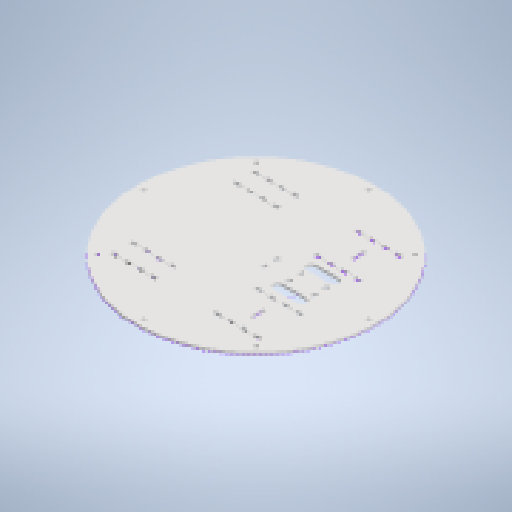
# Autodesk Inventor part: Osn. platform
Saved by Autodesk Inventor 2023.1 (Build 271208000, 208)
## iProperties
Created: 2023-03-13
Part Number: Osn. platform
Material: Типовые
Document SubType Name: Modeling
Designer: User
Density: 1 g/cm^3
Appearance: По умолчанию
Author: User
Autodesk Inventor part; units mm, degrees
ref_plane "YZ Plane" through (0, 0, 0) normal (1, 0, 0) x (0, 1, 0)
ref_plane "XZ Plane" through (0, 0, 0) normal (0, 1, 0) x (-1, 0, 0)
ref_plane "XY Plane" through (0, 0, 0) normal (0, 0, 1) x (1, 0, 0)
sketch "Основ. платформа" plane through (0, 0, 0) normal (0, 1, 0) x (-1, 0, 0)
  circle A0 centre (0, 0) radius 240
  dimension "d117" = 480
  constraints: 1 centre point, 1 coincident
  measures "d117" diameter of A0
extrude "Осн. платформа" add sketch "Основ. платформа" along normal blind 5
sketch "Эскиз14" plane through (0, 5, 0) normal (0, 1, 0) x (1, 0, 0)
  line L0 (-295.6598, 0) -> (443.256, 0) construction
  line L1 (137.6204, 61.9298) -> (150.9061, 61.9298)
  line L2 (150.9061, 61.9298) -> (150.9061, 55.9298)
  line L3 (137.6204, 55.9298) -> (150.9061, 55.9298)
  line L4 (137.6204, 61.9298) -> (137.6204, 55.9298)
  line L5 (111.049, 61.9298) -> (124.3347, 61.9298)
  line L6 (124.3347, 61.9298) -> (124.3347, 55.9298)
  line L7 (111.049, 55.9298) -> (124.3347, 55.9298)
  line L8 (111.049, 61.9298) -> (111.049, 55.9298)
  line L9 (84.4776, 61.9298) -> (97.7633, 61.9298)
  line L10 (97.7633, 61.9298) -> (97.7633, 55.9298)
  line L11 (84.4776, 55.9298) -> (97.7633, 55.9298)
  line L12 (84.4776, 61.9298) -> (84.4776, 55.9298)
  line L13 (57.9061, 144.9298) -> (71.1919, 144.9298)
  line L14 (71.1919, 144.9298) -> (71.1919, 138.9298)
  line L15 (57.9061, 138.9298) -> (71.1919, 138.9298)
  line L16 (57.9061, 144.9298) -> (57.9061, 138.9298)
  line L17 (84.4776, 144.9298) -> (97.7633, 144.9298)
  line L18 (97.7633, 144.9298) -> (97.7633, 138.9298)
  line L19 (84.4776, 138.9298) -> (97.7633, 138.9298)
  line L20 (84.4776, 144.9298) -> (84.4776, 138.9298)
  line L21 (111.049, 144.9298) -> (124.3347, 144.9298)
  line L22 (124.3347, 144.9298) -> (124.3347, 138.9298)
  line L23 (111.049, 138.9298) -> (124.3347, 138.9298)
  line L24 (111.049, 144.9298) -> (111.049, 138.9298)
  line L25 (137.6204, 144.9298) -> (150.9061, 144.9298)
  line L26 (150.9061, 144.9298) -> (150.9061, 138.9298)
  line L27 (137.6204, 138.9298) -> (150.9061, 138.9298)
  line L28 (137.6204, 144.9298) -> (137.6204, 138.9298)
  line L29 (101.4061, 87.5965) -> (101.4061, 113.2631)
  line L30 (101.4061, 113.2631) -> (107.4061, 113.2631)
  line L31 (107.4061, 113.2631) -> (107.4061, 87.5965)
  line L32 (107.4061, 87.5965) -> (101.4061, 87.5965)
  line L33 (57.9061, 61.9298) -> (71.1919, 61.9298)
  line L34 (71.1919, 61.9298) -> (71.1919, 55.9298)
  line L35 (57.9061, 55.9298) -> (71.1919, 55.9298)
  line L36 (57.9061, 61.9298) -> (57.9061, 55.9298)
  line L37 (-58.1024, 138.9298) -> (-70.9595, 138.9298)
  line L38 (-70.9595, 138.9298) -> (-70.9595, 144.9298)
  line L39 (-58.1024, 144.9298) -> (-70.9595, 144.9298)
  line L40 (-58.1024, 138.9298) -> (-58.1024, 144.9298)
  line L41 (-83.8167, 138.9298) -> (-96.6738, 138.9298)
  line L42 (-96.6738, 138.9298) -> (-96.6738, 144.9298)
  line L43 (-83.8167, 144.9298) -> (-96.6738, 144.9298)
  line L44 (-83.8167, 138.9298) -> (-83.8167, 144.9298)
  line L45 (-109.531, 138.9298) -> (-122.3881, 138.9298)
  line L46 (-122.3881, 138.9298) -> (-122.3881, 144.9298)
  line L47 (-109.531, 144.9298) -> (-122.3881, 144.9298)
  line L48 (-109.531, 138.9298) -> (-109.531, 144.9298)
  line L49 (-135.2452, 138.9298) -> (-148.1024, 138.9298)
  line L50 (-148.1024, 138.9298) -> (-148.1024, 144.9298)
  line L51 (-135.2452, 144.9298) -> (-148.1024, 144.9298)
  line L52 (-135.2452, 138.9298) -> (-135.2452, 144.9298)
  line L53 (-58.1024, 144.9298) -> (-148.1024, 144.9298) construction
  line L54 (-148.1024, 100.7298) -> (-58.1024, 100.7298) construction
  line L55 (137.6204, 138.9298) -> (124.3347, 144.9298) construction
  circle A0 centre (130.9776, 141.9298) radius 1.5
  circle A1 centre (104.2556, 141.9298) radius 1.5
  circle A2 centre (77.5336, 141.9298) radius 1.5
  circle A3 centre (130.9776, 58.9298) radius 1.5
  circle A4 centre (104.2556, 58.9298) radius 1.5
  circle A5 centre (77.5336, 58.9298) radius 1.5
  line L56 (-70.9595, 138.9298) -> (-83.8167, 144.9298) construction
  circle A6 centre (-77.3881, 141.9298) radius 1.5
  circle A7 centre (-103.2571, 141.9298) radius 1.5
  circle A8 centre (-129.1261, 141.9298) radius 1.5
  line L57 (-122.3881, 106.7298) -> (-122.3881, 100.7298)
  line L58 (-109.531, 100.7298) -> (-122.3881, 100.7298)
  line L59 (-109.531, 106.7298) -> (-109.531, 100.7298)
  line L60 (-109.531, 106.7298) -> (-122.3881, 106.7298)
  line L61 (-83.8167, 106.7298) -> (-96.6738, 106.7298)
  line L62 (-70.9595, 106.7298) -> (-70.9595, 100.7298)
  line L63 (-58.1024, 100.7298) -> (-70.9595, 100.7298)
  circle A9 centre (-103.2571, 103.7298) radius 1.5
  circle A10 centre (-129.1261, 103.7298) radius 1.5
  line L64 (-135.2452, 106.7298) -> (-135.2452, 100.7298)
  line L65 (-148.1024, 106.7298) -> (-148.1024, 100.7298)
  line L66 (-135.2452, 100.7298) -> (-148.1024, 100.7298)
  line L67 (-135.2452, 106.7298) -> (-148.1024, 106.7298)
  line L68 (-58.1024, 106.7298) -> (-70.9595, 106.7298)
  line L69 (-58.1024, 106.7298) -> (-58.1024, 100.7298)
  line L70 (-96.6738, 106.7298) -> (-96.6738, 100.7298)
  line L71 (-83.8167, 100.7298) -> (-96.6738, 100.7298)
  line L72 (-83.8167, 106.7298) -> (-83.8167, 100.7298)
  circle A11 centre (-77.3881, 103.7298) radius 1.5
  line L73 (111.049, -61.9298) -> (124.3347, -61.9298)
  line L74 (111.049, -61.9298) -> (111.049, -55.9298)
  line L75 (97.7633, -61.9298) -> (97.7633, -55.9298)
  line L76 (71.1919, -61.9298) -> (71.1919, -55.9298)
  line L77 (57.9061, -61.9298) -> (57.9061, -55.9298)
  line L78 (57.9061, -55.9298) -> (71.1919, -55.9298)
  line L79 (57.9061, -61.9298) -> (71.1919, -61.9298)
  line L80 (107.4061, -87.5965) -> (101.4061, -87.5965)
  line L81 (101.4061, -87.5965) -> (101.4061, -113.2631)
  line L82 (107.4061, -113.2631) -> (107.4061, -87.5965)
  line L83 (57.9061, -138.9298) -> (71.1919, -138.9298)
  line L84 (101.4061, -113.2631) -> (107.4061, -113.2631)
  line L85 (84.4776, -138.9298) -> (97.7633, -138.9298)
  line L86 (84.4776, -144.9298) -> (84.4776, -138.9298)
  line L87 (84.4776, -144.9298) -> (97.7633, -144.9298)
  line L88 (97.7633, -144.9298) -> (97.7633, -138.9298)
  line L89 (111.049, -144.9298) -> (111.049, -138.9298)
  line L90 (111.049, -138.9298) -> (124.3347, -138.9298)
  line L91 (111.049, -144.9298) -> (124.3347, -144.9298)
  line L92 (124.3347, -144.9298) -> (124.3347, -138.9298)
  line L93 (137.6204, -61.9298) -> (150.9061, -61.9298)
  line L94 (150.9061, -61.9298) -> (150.9061, -55.9298)
  line L95 (137.6204, -55.9298) -> (150.9061, -55.9298)
  line L96 (137.6204, -61.9298) -> (137.6204, -55.9298)
  circle A12 centre (130.9776, -58.9298) radius 1.5
  line L97 (137.6204, -144.9298) -> (137.6204, -138.9298)
  line L98 (137.6204, -144.9298) -> (150.9061, -144.9298)
  line L99 (150.9061, -144.9298) -> (150.9061, -138.9298)
  line L100 (137.6204, -138.9298) -> (150.9061, -138.9298)
  line L101 (124.3347, -61.9298) -> (124.3347, -55.9298)
  line L102 (111.049, -55.9298) -> (124.3347, -55.9298)
  line L103 (84.4776, -61.9298) -> (97.7633, -61.9298)
  line L104 (84.4776, -55.9298) -> (97.7633, -55.9298)
  line L105 (84.4776, -61.9298) -> (84.4776, -55.9298)
  line L106 (71.1919, -144.9298) -> (71.1919, -138.9298)
  line L107 (57.9061, -144.9298) -> (71.1919, -144.9298)
  line L108 (57.9061, -144.9298) -> (57.9061, -138.9298)
  line L109 (-58.1024, -100.7298) -> (-70.9595, -100.7298)
  line L110 (-70.9595, -106.7298) -> (-70.9595, -100.7298)
  line L111 (-135.2452, -138.9298) -> (-135.2452, -144.9298)
  line L112 (-135.2452, -138.9298) -> (-148.1024, -138.9298)
  line L113 (-148.1024, -138.9298) -> (-148.1024, -144.9298)
  line L114 (-135.2452, -144.9298) -> (-148.1024, -144.9298)
  line L115 (-96.6738, -138.9298) -> (-96.6738, -144.9298)
  line L116 (-83.8167, -138.9298) -> (-96.6738, -138.9298)
  line L117 (-109.531, -138.9298) -> (-109.531, -144.9298)
  line L118 (-83.8167, -144.9298) -> (-96.6738, -144.9298)
  line L119 (-83.8167, -138.9298) -> (-83.8167, -144.9298)
  circle A13 centre (-129.1261, -141.9298) radius 1.5
  circle A14 centre (-129.1261, -103.7298) radius 1.5
  line L120 (-122.3881, -138.9298) -> (-122.3881, -144.9298)
  line L121 (-122.3881, -106.7298) -> (-122.3881, -100.7298)
  line L122 (-109.531, -144.9298) -> (-122.3881, -144.9298)
  line L123 (-109.531, -100.7298) -> (-122.3881, -100.7298)
  line L124 (-109.531, -138.9298) -> (-122.3881, -138.9298)
  line L125 (-109.531, -106.7298) -> (-122.3881, -106.7298)
  line L126 (-148.1024, -100.7298) -> (-58.1024, -100.7298) construction
  line L127 (-58.1024, -144.9298) -> (-148.1024, -144.9298) construction
  line L128 (-70.9595, -138.9298) -> (-70.9595, -144.9298)
  line L129 (-58.1024, -144.9298) -> (-70.9595, -144.9298)
  line L130 (-109.531, -106.7298) -> (-109.531, -100.7298)
  circle A15 centre (-103.2571, -141.9298) radius 1.5
  line L131 (-135.2452, -106.7298) -> (-135.2452, -100.7298)
  line L132 (-135.2452, -106.7298) -> (-148.1024, -106.7298)
  line L133 (-148.1024, -106.7298) -> (-148.1024, -100.7298)
  line L134 (-135.2452, -100.7298) -> (-148.1024, -100.7298)
  circle A16 centre (77.5336, -58.9298) radius 1.5
  line L135 (-58.1024, -106.7298) -> (-70.9595, -106.7298)
  line L136 (-58.1024, -106.7298) -> (-58.1024, -100.7298)
  line L137 (-58.1024, -138.9298) -> (-70.9595, -138.9298)
  line L138 (-58.1024, -138.9298) -> (-58.1024, -144.9298)
  circle A17 centre (130.9776, -141.9298) radius 1.5
  line L139 (137.6204, -138.9298) -> (124.3347, -144.9298) construction
  circle A18 centre (104.2556, -141.9298) radius 1.5
  circle A19 centre (77.5336, -141.9298) radius 1.5
  circle A20 centre (104.2556, -58.9298) radius 1.5
  line L140 (-70.9595, -138.9298) -> (-83.8167, -144.9298) construction
  circle A21 centre (-77.3881, -141.9298) radius 1.5
  circle A22 centre (-103.2571, -103.7298) radius 1.5
  line L141 (-96.6738, -106.7298) -> (-96.6738, -100.7298)
  line L142 (-83.8167, -100.7298) -> (-96.6738, -100.7298)
  line L143 (-83.8167, -106.7298) -> (-83.8167, -100.7298)
  line L144 (-83.8167, -106.7298) -> (-96.6738, -106.7298)
  circle A23 centre (-77.3881, -103.7298) radius 1.5
  point P0 (0, 0)
  point P1 (-58.1024, 122.8298)
  point P2 (-148.1024, 122.8298)
  point P3 (-148.1024, 100.7298)
  point P4 (-148.1024, -122.8298)
  point P5 (-58.1024, -122.8298)
  point P6 (-148.1024, -100.7298)
  constraints: 290 end point, 85 symmetric about line, 24 centre point, 1 horizontal, 12 other
extrude "Выдавливание9" cut sketch "Эскиз14" against normal up to surface (5 mm away)
sketch "Эскиз13" plane through (0, 0, 0) normal (0, -1, 0) x (1, 0, 0)
  line L0 (0, 0) -> (172.9676, 166.3798) construction
  circle A0 centre (0, 0) radius 240 construction
  line L1 (0, 240) -> (240, 0) construction
  line L2 (104.4061, 0) -> (104.4061, 216.1003) construction
  line L3 (107.4061, 87.5961) -> (101.4061, 87.5961) construction
  line L4 (101.4061, 87.5961) -> (101.4061, 113.2631) construction
  line L5 (101.4061, 113.2631) -> (107.4061, 113.2631) construction
  line L6 (107.4061, 113.2631) -> (107.4061, 87.5961) construction
  line L7 (132.4776, 138.9298) -> (132.4776, 144.9298) construction
  line L8 (132.4776, 144.9298) -> (137.6204, 144.9298) construction
  line L9 (137.6204, 144.9298) -> (150.9061, 144.9298) construction
  line L10 (150.9061, 144.9298) -> (150.9061, 138.9298) construction
  line L11 (150.9061, 138.9298) -> (137.6204, 138.9298) construction
  line L12 (137.6204, 138.9298) -> (132.4776, 138.9298) construction
  line L13 (137.6204, 138.9298) -> (137.6204, 144.9298) construction
  line L14 (101.4061, 144.9298) -> (101.4061, 138.9298) construction
  line L15 (101.4061, 138.9298) -> (97.7633, 138.9298) construction
  line L16 (97.7633, 144.9298) -> (97.7633, 138.9298) construction
  line L17 (84.4776, 144.9298) -> (97.7633, 144.9298) construction
  line L18 (84.4776, 138.9298) -> (84.4776, 144.9298) construction
  line L19 (84.4776, 138.9298) -> (79.3347, 138.9298) construction
  line L20 (79.3347, 138.9298) -> (79.3347, 144.9298) construction
  line L21 (79.3347, 144.9298) -> (84.4776, 144.9298) construction
  line L22 (97.7633, 144.9298) -> (101.4061, 144.9298) construction
  line L23 (97.7633, 138.9298) -> (84.4776, 138.9298) construction
  line L24 (107.4061, 138.9298) -> (107.4061, 144.9298) construction
  line L25 (107.4061, 144.9298) -> (111.049, 144.9298) construction
  line L26 (111.049, 144.9298) -> (124.3347, 144.9298) construction
  line L27 (124.3347, 144.9298) -> (129.4776, 144.9298) construction
  line L28 (129.4776, 144.9298) -> (129.4776, 138.9298) construction
  line L29 (129.4776, 138.9298) -> (124.3347, 138.9298) construction
  line L30 (124.3347, 138.9298) -> (111.049, 138.9298) construction
  line L31 (111.049, 138.9298) -> (107.4061, 138.9298) construction
  line L32 (111.049, 138.9298) -> (111.049, 144.9298) construction
  line L33 (124.3347, 144.9298) -> (124.3347, 138.9298) construction
  line L34 (57.9061, 144.9298) -> (71.1919, 144.9298) construction
  line L35 (71.1919, 144.9298) -> (76.3347, 144.9298) construction
  line L36 (76.3347, 144.9298) -> (76.3347, 138.9298) construction
  line L37 (76.3347, 138.9298) -> (71.1919, 138.9298) construction
  line L38 (71.1919, 138.9298) -> (57.9061, 138.9298) construction
  line L39 (57.9061, 138.9298) -> (57.9061, 144.9298) construction
  line L40 (71.1919, 144.9298) -> (71.1919, 138.9298) construction
  circle A1 centre (0, 0) radius 240 construction
  line L41 (150.9061, -55.9298) -> (137.6204, -55.9298)
  line L42 (137.6204, -55.9298) -> (137.6204, -61.9298)
  line L43 (137.6204, -61.9298) -> (150.9061, -61.9298)
  line L44 (150.9061, -61.9298) -> (150.9061, -55.9298)
  line L45 (71.1919, -144.9298) -> (71.1919, -138.9298)
  line L46 (71.1919, -138.9298) -> (57.9061, -138.9298)
  line L47 (57.9061, -138.9298) -> (57.9061, -144.9298)
  line L48 (57.9061, -144.9298) -> (71.1919, -144.9298)
  line L49 (107.4061, 113.2631) -> (101.4061, 113.2631) construction
  line L50 (101.4061, 113.2631) -> (101.4061, 87.5965) construction
  line L51 (101.4061, 87.5965) -> (107.4061, 87.5965) construction
  line L52 (107.4061, 87.5965) -> (107.4061, 113.2631) construction
  line L53 (111.049, 144.9298) -> (111.049, 138.9298) construction
  line L54 (111.049, 138.9298) -> (124.3347, 138.9298) construction
  line L55 (124.3347, 138.9298) -> (124.3347, 144.9298) construction
  line L56 (124.3347, 144.9298) -> (111.049, 144.9298) construction
  line L57 (97.7633, 144.9298) -> (84.4776, 144.9298) construction
  line L58 (84.4776, 144.9298) -> (84.4776, 138.9298) construction
  line L59 (84.4776, 138.9298) -> (97.7633, 138.9298) construction
  line L60 (97.7633, 138.9298) -> (97.7633, 144.9298) construction
  line L61 (137.6204, -138.9298) -> (137.6204, -144.9298)
  line L62 (137.6204, -144.9298) -> (150.9061, -144.9298)
  line L63 (150.9061, -144.9298) -> (150.9061, -138.9298)
  line L64 (150.9061, -138.9298) -> (137.6204, -138.9298)
  line L65 (107.4061, -113.2631) -> (107.4061, -87.5965)
  line L66 (107.4061, -87.5965) -> (101.4061, -87.5965)
  line L67 (101.4061, -87.5965) -> (101.4061, -113.2631)
  line L68 (101.4061, -113.2631) -> (107.4061, -113.2631)
  line L69 (124.3347, -55.9298) -> (111.049, -55.9298)
  line L70 (111.049, -55.9298) -> (111.049, -61.9298)
  line L71 (111.049, -61.9298) -> (124.3347, -61.9298)
  line L72 (124.3347, -61.9298) -> (124.3347, -55.9298)
  line L73 (84.4776, -138.9298) -> (84.4776, -144.9298)
  line L74 (84.4776, -144.9298) -> (97.7633, -144.9298)
  line L75 (97.7633, -144.9298) -> (97.7633, -138.9298)
  line L76 (97.7633, -138.9298) -> (84.4776, -138.9298)
  line L77 (57.9061, -55.9298) -> (57.9061, -61.9298)
  line L78 (57.9061, -61.9298) -> (71.1919, -61.9298)
  line L79 (71.1919, -61.9298) -> (71.1919, -55.9298)
  line L80 (71.1919, -55.9298) -> (57.9061, -55.9298)
  line L81 (150.9061, 144.9298) -> (137.6204, 144.9298) construction
  line L82 (137.6204, 144.9298) -> (137.6204, 138.9298) construction
  line L83 (137.6204, 138.9298) -> (150.9061, 138.9298) construction
  line L84 (150.9061, 138.9298) -> (150.9061, 144.9298) construction
  line L85 (57.9061, 144.9298) -> (57.9061, 138.9298) construction
  line L86 (57.9061, 138.9298) -> (71.1919, 138.9298) construction
  line L87 (71.1919, 138.9298) -> (71.1919, 144.9298) construction
  line L88 (71.1919, 144.9298) -> (57.9061, 144.9298) construction
  line L89 (111.049, -144.9298) -> (124.3347, -144.9298)
  line L90 (124.3347, -144.9298) -> (124.3347, -138.9298)
  line L91 (124.3347, -138.9298) -> (111.049, -138.9298)
  line L92 (111.049, -138.9298) -> (111.049, -144.9298)
  line L93 (97.7633, -55.9298) -> (84.4776, -55.9298)
  line L94 (84.4776, -55.9298) -> (84.4776, -61.9298)
  line L95 (84.4776, -61.9298) -> (97.7633, -61.9298)
  line L96 (97.7633, -61.9298) -> (97.7633, -55.9298)
  line L97 (0, -35.6359) -> (0, 40.5263) construction
  line L98 (0, 0) -> (-172.9676, 166.3798) construction
  line L99 (0, 240) -> (-240, 0) construction
  line L100 (-104.4061, 0) -> (-104.4061, 216.1003) construction
  line L101 (-107.4061, 87.5961) -> (-101.4061, 87.5961) construction
  line L102 (-101.4061, 87.5961) -> (-101.4061, 113.2631) construction
  line L103 (-101.4061, 113.2631) -> (-107.4061, 113.2631) construction
  line L104 (-107.4061, 113.2631) -> (-107.4061, 87.5961) construction
  line L105 (-132.4776, 138.9298) -> (-132.4776, 144.9298) construction
  line L106 (-132.4776, 144.9298) -> (-137.6204, 144.9298) construction
  line L107 (-137.6204, 144.9298) -> (-150.9061, 144.9298) construction
  line L108 (-150.9061, 144.9298) -> (-150.9061, 138.9298) construction
  line L109 (-150.9061, 138.9298) -> (-137.6204, 138.9298) construction
  line L110 (-137.6204, 138.9298) -> (-132.4776, 138.9298) construction
  line L111 (-137.6204, 138.9298) -> (-137.6204, 144.9298) construction
  line L112 (-101.4061, 144.9298) -> (-101.4061, 138.9298) construction
  line L113 (-101.4061, 138.9298) -> (-97.7633, 138.9298) construction
  line L114 (-97.7633, 144.9298) -> (-97.7633, 138.9298) construction
  line L115 (-84.4776, 144.9298) -> (-97.7633, 144.9298) construction
  line L116 (-84.4776, 138.9298) -> (-84.4776, 144.9298) construction
  line L117 (-84.4776, 138.9298) -> (-79.3347, 138.9298) construction
  line L118 (-79.3347, 138.9298) -> (-79.3347, 144.9298) construction
  line L119 (-79.3347, 144.9298) -> (-84.4776, 144.9298) construction
  line L120 (-97.7633, 144.9298) -> (-101.4061, 144.9298) construction
  line L121 (-97.7633, 138.9298) -> (-84.4776, 138.9298) construction
  line L122 (-107.4061, 138.9298) -> (-107.4061, 144.9298) construction
  line L123 (-107.4061, 144.9298) -> (-111.049, 144.9298) construction
  line L124 (-111.049, 144.9298) -> (-124.3347, 144.9298) construction
  line L125 (-124.3347, 144.9298) -> (-129.4776, 144.9298) construction
  line L126 (-129.4776, 144.9298) -> (-129.4776, 138.9298) construction
  line L127 (-129.4776, 138.9298) -> (-124.3347, 138.9298) construction
  line L128 (-124.3347, 138.9298) -> (-111.049, 138.9298) construction
  line L129 (-111.049, 138.9298) -> (-107.4061, 138.9298) construction
  line L130 (-111.049, 138.9298) -> (-111.049, 144.9298) construction
  line L131 (-124.3347, 144.9298) -> (-124.3347, 138.9298) construction
  line L132 (-57.9061, 144.9298) -> (-71.1919, 144.9298) construction
  line L133 (-71.1919, 144.9298) -> (-76.3347, 144.9298) construction
  line L134 (-76.3347, 144.9298) -> (-76.3347, 138.9298) construction
  line L135 (-76.3347, 138.9298) -> (-71.1919, 138.9298) construction
  line L136 (-71.1919, 138.9298) -> (-57.9061, 138.9298) construction
  line L137 (-57.9061, 138.9298) -> (-57.9061, 144.9298) construction
  line L138 (-71.1919, 144.9298) -> (-71.1919, 138.9298) construction
  line L139 (-107.4061, 113.2631) -> (-101.4061, 113.2631) construction
  line L140 (-101.4061, 113.2631) -> (-101.4061, 87.5965) construction
  line L141 (-101.4061, 87.5965) -> (-107.4061, 87.5965) construction
  line L142 (-107.4061, 87.5965) -> (-107.4061, 113.2631) construction
  line L143 (-111.049, 144.9298) -> (-111.049, 138.9298) construction
  line L144 (-111.049, 138.9298) -> (-124.3347, 138.9298) construction
  line L145 (-124.3347, 138.9298) -> (-124.3347, 144.9298) construction
  line L146 (-124.3347, 144.9298) -> (-111.049, 144.9298) construction
  line L147 (-97.7633, 144.9298) -> (-84.4776, 144.9298) construction
  line L148 (-84.4776, 144.9298) -> (-84.4776, 138.9298) construction
  line L149 (-84.4776, 138.9298) -> (-97.7633, 138.9298) construction
  line L150 (-97.7633, 138.9298) -> (-97.7633, 144.9298) construction
  line L151 (-150.9061, 144.9298) -> (-137.6204, 144.9298) construction
  line L152 (-137.6204, 144.9298) -> (-137.6204, 138.9298) construction
  line L153 (-137.6204, 138.9298) -> (-150.9061, 138.9298) construction
  line L154 (-150.9061, 138.9298) -> (-150.9061, 144.9298) construction
  line L155 (-57.9061, 144.9298) -> (-57.9061, 138.9298) construction
  line L156 (-57.9061, 138.9298) -> (-71.1919, 138.9298) construction
  line L157 (-71.1919, 138.9298) -> (-71.1919, 144.9298) construction
  line L158 (-71.1919, 144.9298) -> (-57.9061, 144.9298) construction
  point P0 (104.4061, 100.4296)
  point P1 (-104.4061, 100.4296)
  dimension "d121" = 25.667
  constraints: 318 end point, 39 symmetric about line, 21 horizontal, 16 vertical, 4 point on circle, 2 parallel, 1 centre point, 1 perpendicular, 28 other
  measures "d121" distance of L3.end L4.end
sketch "Эскиз16" plane through (0, 5, 0) normal (0, 1, 0) x (1, 0, 0)
  line L0 (-17, -32) -> (-7, -32) construction
  line L1 (-7, -32) -> (-7, -25) construction
  line L2 (-7, -25) -> (-17, -25) construction
  line L3 (-17, -25) -> (-17, -32) construction
  line L4 (66.5859, 0) -> (-61.9521, 0) construction
  line L5 (0, -82.102) -> (0, 52.9941) construction
  line L6 (-17, -75) -> (-17, -82) construction
  line L7 (-17, -82) -> (-7, -82) construction
  line L8 (-7, -82) -> (-7, -75) construction
  line L9 (-7, -75) -> (-17, -75) construction
  line L10 (-17, -125) -> (-17, -132) construction
  line L11 (-17, -132) -> (-7, -132) construction
  line L12 (-7, -132) -> (-7, -125) construction
  line L13 (-7, -125) -> (-17, -125) construction
  line L14 (7, -25) -> (7, -32) construction
  line L15 (7, -32) -> (17, -32) construction
  line L16 (17, -32) -> (17, -25) construction
  line L17 (17, -25) -> (7, -25) construction
  line L18 (7, -75) -> (7, -82) construction
  line L19 (7, -82) -> (17, -82) construction
  line L20 (17, -82) -> (17, -75) construction
  line L21 (17, -75) -> (7, -75) construction
  line L22 (7, -125) -> (7, -132) construction
  line L23 (7, -132) -> (17, -132) construction
  line L24 (17, -132) -> (17, -125) construction
  line L25 (17, -125) -> (7, -125) construction
  line L26 (32, -7) -> (25, -7)
  line L27 (25, -7) -> (25, -17)
  line L28 (25, -17) -> (32, -17)
  line L29 (32, -17) -> (32, -7)
  line L30 (32, -7) -> (25, -17) construction
  line L31 (25, -7) -> (32, -17) construction
  line L32 (75, -17) -> (82, -17)
  line L33 (82, -17) -> (82, -7)
  line L34 (82, -7) -> (75, -7)
  line L35 (75, -7) -> (75, -17)
  line L36 (125, -17) -> (132, -17)
  line L37 (132, -17) -> (132, -7)
  line L38 (132, -7) -> (125, -7)
  line L39 (125, -7) -> (125, -17)
  line L40 (25, 7) -> (32, 7)
  line L41 (32, 7) -> (32, 17)
  line L42 (32, 17) -> (25, 17)
  line L43 (25, 17) -> (25, 7)
  line L44 (75, 7) -> (82, 7)
  line L45 (82, 7) -> (82, 17)
  line L46 (82, 17) -> (75, 17)
  line L47 (75, 17) -> (75, 7)
  line L48 (125, 7) -> (132, 7)
  line L49 (132, 7) -> (132, 17)
  line L50 (132, 17) -> (125, 17)
  line L51 (125, 17) -> (125, 7)
  circle A0 centre (104.2556, -58.9298) radius 1.5 construction
  circle A1 centre (130.9776, -58.9298) radius 1.5 construction
  line L52 (125.6303, -33.4298) -> (77.5364, -33.4298) construction
  line L53 (125.6303, -24.4298) -> (77.5364, -24.4298)
  line L54 (77.5364, -42.4298) -> (125.6303, -42.4298)
  arc A2 (125.6303, -42.4298) -> (125.6303, -24.4298) centre (125.6303, -33.4298) ccw
  arc A3 (77.5364, -24.4298) -> (77.5364, -42.4298) centre (77.5364, -33.4298) ccw
  line L55 (125.6303, 33.4298) -> (77.5364, 33.4298) construction
  line L56 (125.6303, 24.4298) -> (77.5364, 24.4298)
  line L57 (77.5364, 42.4298) -> (125.6303, 42.4298)
  arc A4 (125.6303, 24.4298) -> (125.6303, 42.4298) centre (125.6303, 33.4298) ccw
  arc A5 (77.5364, 42.4298) -> (77.5364, 24.4298) centre (77.5364, 33.4298) ccw
  circle A6 centre (-225.3213, 0) radius 4
  circle A7 centre (-159.3262, -159.3262) radius 4
  circle A8 centre (0, -225.3213) radius 4
  circle A9 centre (159.3262, -159.3262) radius 4
  circle A10 centre (225.3213, 0) radius 4
  circle A11 centre (159.3262, 159.3262) radius 4
  circle A12 centre (0, 225.3213) radius 4
  circle A13 centre (-159.3262, 159.3262) radius 4
  line L58 (-22, 32) -> (22, 32) construction
  line L59 (32, 22) -> (32, -22) construction
  line L60 (22, -32) -> (-22, -32) construction
  line L61 (-32, -22) -> (-32, 22) construction
  line L62 (-32, 32) -> (32, -32) construction
  line L63 (32, 32) -> (-32, -32) construction
  arc A14 (-22, 32) -> (-32, 22) centre (-22, 22) ccw construction
  arc A15 (-32, -22) -> (-22, -32) centre (-22, -22) ccw construction
  arc A16 (22, -32) -> (32, -22) centre (22, -22) ccw construction
  arc A17 (32, 22) -> (22, 32) centre (22, 22) ccw construction
  point P0 (0, 0)
  point P1 (-7, -28.5)
  point P2 (-7, -78.5)
  point P3 (-7, -128.5)
  point P4 (17, -28.5)
  point P5 (17, -78.5)
  point P6 (17, -128.5)
  point P7 (28.5, -12)
  point P8 (25, -12)
  point P9 (28.5, -7)
  point P10 (78.5, -7)
  point P11 (75, -12)
  point P12 (128.5, -7)
  point P13 (125, -12)
  point P14 (28.5, 17)
  point P15 (25, 12)
  point P16 (78.5, 17)
  point P17 (75, 12)
  point P18 (128.5, 17)
  point P19 (125, 12)
  point P20 (101.5834, -33.4298)
  point P21 (101.5834, 33.4298)
  dimension "d160" = 50
  dimension "d163" = 24
  dimension "d166" = 7
  dimension "d167" = 10
  dimension "d168" = 25
  dimension "d169" = 7
  dimension "d172" = 50
  dimension "d175" = 24
  dimension "d178" = 18
  dimension "d179" = 15
  dimension "d182" = 8
  dimension "d185" = 360
  dimension "d189" = 10
  constraints: 132 end point, 16 centre point, 16 point on circle, 12 tangent, 8 midpoint, 8 point on line, 7 horizontal, 7 symmetric about line, 5 parallel, 4 vertical, 3 equal radius, 2 perpendicular, 114 other
  measures "d160" distance of L2.end L6.start
  measures "d163" distance of L2.end L14.start
  measures "d166" distance of L28.end L27.end
  measures "d167" distance of L27.end L26.end
  measures "d168" distance from line of L5 point (25, -12)
  measures "d169" distance from line of L4 point (28.5, -7)
  measures "d172" distance of L27.end L32.start
  measures "d175" distance of L27.end L40.start
  measures "d178" diameter of A3
  measures "d179" distance edge to line of A0 L54
  measures "d182" diameter of A6
  measures "d189" radius of A14
extrude "Выдавливание10" cut sketch "Эскиз16" against normal blind 10
